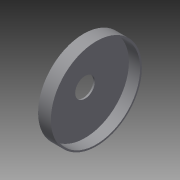
# Autodesk Inventor part: Ground_shield_v2
Saved by Autodesk Inventor 2014 SP1 (Build 180222100, 222)
## iProperties
Created: 2012-06-12
Part Number: Ground_shield_v2
Material: Steel, Chrome Plated
Document SubType Name: Sheet Metal
Designer: Breckenridge2 User
Density: 1 g/cm^3
Sheet Metal Rule: Default
Appearance: Chrome - Polished
Author: Breckenridge2 User
Autodesk Inventor part; units mm, degrees
ref_plane "YZ Plane" through (0, 0, 0) normal (1, 0, 0) x (0, 1, 0)
ref_plane "XZ Plane" through (0, 0, 0) normal (0, 1, 0) x (-1, 0, 0)
ref_plane "XY Plane" through (0, 0, 0) normal (0, 0, 1) x (1, 0, 0)
sketch "Sketch1" plane through (0, 0, 0) normal (1, 0, 0) x (0, 1, 0)
  circle A0 centre (0, -0.3053) radius 87.63
  point P0 (0, 0)
  dimension "d0" = 175.26
  constraints: 1 centre point
  measures "d0" diameter of A0
extrude "Extrusion1" add sketch "Sketch1" along normal blind 24.638
sketch "Sketch2" plane through (24.638, 0, -0.3053) normal (1, 0, 0) x (0, 0, -1)
  circle A0 centre (-0.3053, 0) radius 84.455
  dimension "d3" = 168.91
  constraints: 1 centre point, 1 coincident
  measures "d3" diameter of A0
extrude "Cut1" cut sketch "Sketch2" against normal blind 21.59
sketch "Sketch3" plane through (3.048, 0, 0) normal (1, 0, 0) x (0, 0, -1)
  circle A0 centre (0, 0) radius 84.455 projected
  circle A1 centre (0, 0) radius 19.05
  dimension "d6" = 38.1
  constraints: 1 centre point, 1 coincident
  measures "d6" diameter of A1
extrude "Cut2" cut sketch "Sketch3" against normal up to next contours A1
equation "\"d7\" = Thickness"
equation "\"BendRadius\" = Thickness"
equation "\"BendReliefWidth\" = Thickness"
equation "\"BendReliefDepth\" = 0.5 * Thickness"
equation "\"CornerReliefSize\" = 4 * Thickness"
equation "\"MinimumRemnant\" = 2 * Thickness"
equation "\"TransitionRadius\" = BendRadius"
equation "\"JacobiRadiusSize\" = BendRadius"
equation "\"GapSize\" = Thickness"
equation "\"Thickness\" = 3.048"
body "Solid1"
